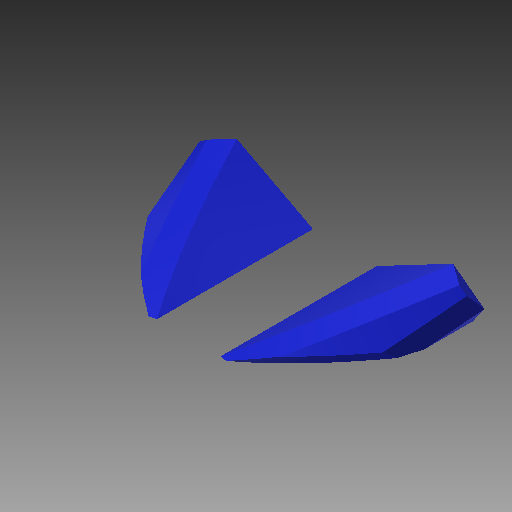
# Autodesk Inventor part: Eyes
Saved by Autodesk Inventor 2017.2 (Build 212233000, 233)
## iProperties
Created: 2014-01-19
Part Number: Eyes
Material: Generic
Document SubType Name: Modeling
Designer: Spooner
Density: 1 g/cm^3
Appearance: Blue - Wall Paint - Glossy
Mass: 0.0244767 g
Surface Area: 0.919147 cm^2
Volume: 0.0244767 cm^3
Author: Spooner
Autodesk Inventor part; units mm, degrees
ref_plane "XZ Plane" through (0, 0, 0) normal (0, 1, 0) x (-1, 0, 0)
ref_plane "XY Plane" through (0, 0, 0) normal (0, 0, 1) x (1, 0, 0)
sketch "Sketch1" plane through (0, 0, 0) normal (1, 0, 0) x (0, 1, 0)
  line L0 (-6.35, 0) -> (-5.6104, 2.032)
  line L1 (-5.6104, 2.032) -> (5.6104, 2.032)
  line L2 (5.6104, 2.032) -> (6.35, 0)
  line L3 (6.35, 0) -> (1.997, -3.048)
  line L4 (1.997, -3.048) -> (-1.997, -3.048)
  line L5 (-1.997, -3.048) -> (-6.35, 0)
  point P0 (0, 0)
  point P1 (0, 2.032)
  dimension "d0" = 110
  dimension "d1" = 110
  dimension "d2" = 145
  dimension "d3" = 5.08
  dimension "d4" = 12.7
  dimension "d6" = 2.032
  constraints: 12 end point, 2 equal length, 1 horizontal, 1 horizontal alignment, 1 midpoint, 1 parallel, 1 vertical alignment
  measures "d0" angle of L1 L0
  measures "d1" angle of L2 L1
  measures "d2" angle of L4 L5
  measures "d3" distance between parallel lines of L4 L1
  measures "d4" distance of L2.end L0.start
  measures "d6" distance from line of point (0, 0) L1
ref_plane "Work Plane1" through (13.97, 0, 0) normal (1, 0, 0) x (0, 1, 0)
sketch "Sketch2" plane through (13.97, 0, 0) normal (1, 0, 0) x (0, 1, 0)
  line L0 (-12.7, 0) -> (-11.7848, 1.9627)
  line L1 (-11.7848, 1.9627) -> (0, 11.8513)
  line L2 (0, 11.8513) -> (0, 11.8513)
  line L3 (0, 11.8513) -> (11.7848, 1.9627)
  line L4 (11.7848, 1.9627) -> (12.7, 0)
  line L5 (12.7, 0) -> (4.191, -4.9127)
  line L6 (4.191, -4.9127) -> (-4.191, -4.9127)
  line L7 (-4.191, -4.9127) -> (-12.7, 0)
  point P0 (0, 0)
  point P1 (0, -4.9127)
  point P2 (0, 11.8513)
  dimension "d8" = 150
  dimension "d9" = 150
  dimension "d14" = 8.382
  dimension "d15" = 16.764
  dimension "d22" = 25.4
  dimension "d26" = 155
  dimension "d28" = 155
  dimension "d29" = 0
  dimension "d30" = 140
  dimension "d31" = 140
  constraints: 16 end point, 2 horizontal alignment, 2 midpoint, 2 vertical alignment, 1 horizontal, 1 parallel
  measures "d8" angle of L6 L7
  measures "d9" angle of L5 L6
  measures "d14" distance of L5.end L6.end
  measures "d15" distance between parallel lines of L6 L2
  measures "d22" distance of L4.end L0.start
  measures "d26" angle of L0 L1
  measures "d28" angle of L4 L3
  measures "d29" distance of L1.end L2.end
  measures "d30" angle of L2 L1
  measures "d31" angle of L3 L2
loft "Main Body" add profiles "Sketch1", "Sketch2"
sketch "Sketch3" plane through (0, -5.6104, 2.032) normal (-1, 0, 0) x (0, 0, 1)
  line L0 (0, 5.6104) -> (0, 11.2208) projected
  line L1 (-5.08, 7.6074) -> (-5.08, 3.6134) projected
  line L2 (-5.08, 3.6134) -> (-2.032, -0.7396) projected
  line L3 (4.445, 12.0243) -> (4.445, 10.5003)
  line L4 (4.445, 10.5003) -> (2.54, 6.8804)
  line L5 (2.54, 6.8804) -> (2.54, 10.6904)
  line L6 (2.54, 10.6904) -> (4.445, 12.0243)
  line L7 (0, 5.6104) -> (9.8193, 5.6104) projected
  line L8 (4.445, -0.8035) -> (4.445, 0.7205)
  line L9 (4.445, 0.7205) -> (2.54, 4.3404)
  line L10 (2.54, 4.3404) -> (2.54, 0.5304)
  line L11 (2.54, 0.5304) -> (4.445, -0.8035)
  point P0 (-2.032, 5.6104)
  dimension "d32" = 1.905
  dimension "d33" = 3.81
  dimension "d34" = 1.524
  dimension "d35" = 2.54
  dimension "d36" = 1.27
  constraints: 16 end point, 4 symmetric about line, 1 parallel, 1 perpendicular, 1 vertical
  measures "d32" distance between parallel lines of L5 L3
  measures "d33" distance of L4.end L5.end
  measures "d34" distance of L3.start L3.end
  measures "d35" distance between parallel lines of L0 L5
  measures "d36" vertical distance of point (-2.032, 5.61) L4.end
extrude "Create Eyes" cut sketch "Sketch3" against normal blind 11.43 keep common part
chamfer "Eyes Chamfer" distance 0.508 angle 45 8 edges at (7.7963, 3.1773, 5.5757) (11.43, 5.3124, 6.0348) (9.7825, 5.4541, 5.1062) (6.0686, 3.3311, 4.572) (7.7795, -3.1692, 5.5715) (6.0907, -3.3528, 4.572) (9.7825, -5.4541, 5.1062) (11.43, -5.3124, 6.0348)
equation "\"d1\" = d0"
equation "\"d9\" = d8"
equation "\"d28\" = d26"
equation "\"d31\" = d30"
body "Solid1"
